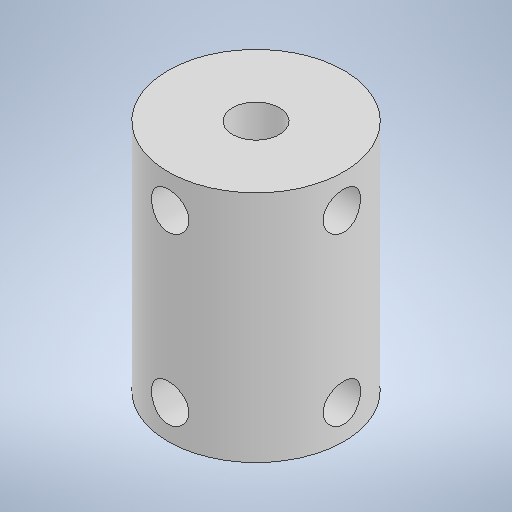
# Autodesk Inventor part: Shaft coupler
Saved by Autodesk Inventor 2025.2 (Build 292293000, 293)
## iProperties
Created: 2025-01-27
Part Number: Shaft coupler
Material: Generic
Document SubType Name: Modeling
Designer: caomi
Density: 1 g/cm^3
Appearance: Default
Author: caomi
Autodesk Inventor part; units mm, degrees
ref_plane "YZ Plane" through (0, 0, 0) normal (1, 0, 0) x (0, 1, 0)
ref_plane "XZ Plane" through (0, 0, 0) normal (0, 1, 0) x (-1, 0, 0)
sketch "Sketch1" plane through (0, 0, 0) normal (0, 1, 0) x (-1, 0, 0)
  circle A0 centre (0, 0) radius 9.4
  circle A1 centre (0, 0) radius 4
  circle A2 centre (0, 0) radius 2.5
  dimension "d0" = 8
  dimension "d1" = 18.8
  dimension "d2" = 5
  constraints: 3 centre point, 3 coincident
  measures "d0" diameter of A1
  measures "d1" diameter of A0
  measures "d2" diameter of A2
extrude "Extrusion1" add sketch "Sketch1" along normal blind 25 contours A0 | A1
extrude "Extrusion2" cut sketch "Sketch1" along normal blind 18.5 contours A1
ref_plane "Work Plane1" through (0, 0, 9.4) normal (0, 0, 1) x (1, 0, 0)
sketch "Sketch2" plane through (0, 0, 9.4) normal (0, 0, 1) x (1, 0, 0)
  circle A0 centre (0, 21.4) radius 2
  circle A1 centre (0, 3.6) radius 2
  line L0 (9.4, 0) -> (-9.4, 0) projected
  line L1 (9.4, 25) -> (-9.4, 25) projected
  point P0 (0, 0)
  dimension "d7" = 4
  dimension "d8" = 3.6
  dimension "d9" = 3.6
  constraints: 2 centre point, 2 vertical alignment, 1 equal radius
  measures "d7" diameter of A0
  measures "d8" distance from line of A1.centre L0
  measures "d9" distance from line of L1 A0.centre
extrude "Extrusion3" cut sketch "Sketch2" against normal up to next
pattern_circular "Circular Pattern1" count 2 over 90 about axis through (0, 0, 0) along (0, 1, 0) of "Extrusion3"
equation "\"d9\" = d8"
body "Solid1"
